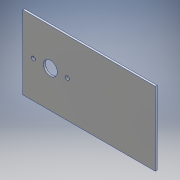
# Autodesk Inventor part: sholder_2
Saved by Autodesk Inventor 2016 (Build 200138000, 138)
## iProperties
Created: 2016-06-28
Part Number: sholder_2
Material: アルミニウム 6061
Document SubType Name: Modeling
Designer: 宏太
Density: 2.7 g/cm^3
Appearance: アルミニウム - フラット
Mass: 272.064 g
Surface Area: 296.193 cm^2
Volume: 100.765 cm^3
Author: 宏太
Autodesk Inventor part; units mm, degrees
ref_plane "YZ Plane" through (0, 0, 0) normal (1, 0, 0) x (0, 1, 0)
ref_plane "XZ Plane" through (0, 0, 0) normal (0, 1, 0) x (-1, 0, 0)
ref_plane "XY Plane" through (0, 0, 0) normal (0, 0, 1) x (1, 0, 0)
sketch "スケッチ1" plane through (0, 0, 0) normal (0, 1, 0) x (-1, 0, 0)
  line L0 (-70, 40) -> (70, 40)
  line L1 (70, 40) -> (70, -40)
  line L2 (70, -40) -> (-70, -40)
  line L3 (-70, -40) -> (-70, 40)
  line L4 (-70, 40) -> (70, -40) construction
  line L5 (70, 40) -> (-70, -40) construction
  point P0 (0, 0)
  dimension "d0" = 140
  dimension "d1" = 80
  constraints: 12 end point, 2 midpoint, 2 parallel, 1 horizontal, 1 perpendicular
  measures "d0" distance of L1.end L2.end
  measures "d1" distance of L0.end L1.end
extrude "押し出し1" add sketch "スケッチ1" along normal blind 2
sketch "スケッチ2" plane through (0, 2, 0) normal (0, 1, 0) x (1, 0, 0)
  circle A0 centre (-40, 0) radius 7.5
  circle A1 centre (-58.5, 0) radius 2.1
  circle A2 centre (-21.5, 0) radius 2.1
  line L0 (70, 40) -> (70, -40) projected
  point P0 (0, 0)
  dimension "d4" = 15
  dimension "d6" = 4.2
  dimension "d7" = 4.2
  dimension "d8" = 37
  dimension "d9" = 18.5
  dimension "d12" = 110
  constraints: 3 centre point
  measures "d4" diameter of A0
  measures "d6" diameter of A1
  measures "d7" diameter of A2
  measures "d8" distance of A2.centre A1.centre
  measures "d9" distance of A0.centre A1.centre
  measures "d12" distance from line of L0 A0.centre
extrude "押し出し2" cut sketch "スケッチ2" against normal blind 8
sketch "スケッチ3" plane through (70, 0, 40) normal (1, 0, 0) x (0, 0, -1)
  line L0 (0, 2) -> (80, 2) projected
  line L1 (0, 0) -> (80, 0)
  line L2 (80, 0) -> (80, 2)
  line L3 (80, 2) -> (0, 2)
  line L4 (0, 2) -> (0, 0)
  point P0 (40, 0)
  constraints: 8 end point, 2 parallel, 1 horizontal, 1 perpendicular
extrude "押し出し3" add sketch "スケッチ3" along normal blind 4
